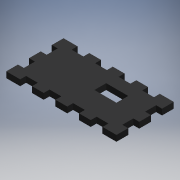
# Autodesk Inventor part: left
Saved by Autodesk Inventor 2019 (Build 230136000, 136)
## iProperties
Created: 2018-06-07
Part Number: left
Material: PBT Plastic Black
Document SubType Name: Modeling
Designer: stra92745
Density: 1.31 g/cm^3
Appearance: Smooth - White
Author: stra92745
Autodesk Inventor part; units mm, degrees
ref_plane "YZ Plane" through (0, 0, 0) normal (1, 0, 0) x (0, 1, 0)
ref_plane "XZ Plane" through (0, 0, 0) normal (0, 1, 0) x (-1, 0, 0)
ref_plane "XY Plane" through (0, 0, 0) normal (0, 0, 1) x (1, 0, 0)
sketch "Sketch1" plane through (0, 0, 0) normal (0, 1, 0) x (-1, 0, 0)
  line L0 (0, 0) -> (-75, 0)
  line L1 (-75, 0) -> (-75, -39)
  line L2 (-75, -39) -> (0, -39)
  line L3 (0, -39) -> (0, 0)
  line L4 (-41, -27) -> (-56, -27)
  line L5 (-56, -27) -> (-56, -19)
  line L6 (-56, -19) -> (-41, -19)
  line L7 (-41, -19) -> (-41, -27)
  dimension "d0" = 75
  dimension "d1" = 39
  dimension "d21" = 15
  dimension "d22" = 19
  dimension "d23" = 8
  dimension "d24" = 19
  constraints: 16 end point, 4 parallel, 2 horizontal, 2 perpendicular
  measures "d0" distance of L2.end L1.end
  measures "d1" distance of L1.end L0.end
  measures "d21" distance of L5.end L6.end
  measures "d22" distance between parallel lines of L1 L5
  measures "d23" distance of L6.end L4.start
  measures "d24" distance between parallel lines of L0 L6
extrude "Extrusion1" add sketch "Sketch1" along normal blind 4
sketch "Sketch2" plane through (0, 4, 0) normal (0, 1, 0) x (1, 0, 0)
  line L0 (0, 39) -> (0, 0) construction
  line L1 (75, 39) -> (0, 39) construction
  line L2 (75, 0) -> (75, 39) construction
  line L3 (0, 0) -> (75, 0) construction
  line L4 (4, 35) -> (4, 4) construction
  line L5 (4, 4) -> (71, 4) construction
  line L6 (71, 4) -> (71, 35) construction
  line L7 (71, 35) -> (4, 35) construction
  line L8 (0, 39) -> (0, 0) construction
  line L9 (0, 19.5) -> (75, 19.5) construction
  line L10 (37.5, 39) -> (37.5, 0) construction
  line L11 (0, 31) -> (4, 31)
  line L12 (4, 31) -> (4, 23.5)
  line L13 (4, 23.5) -> (0, 23.5)
  line L14 (0, 23.5) -> (0, 31)
  line L15 (75, 39) -> (0, 39) projected
  line L16 (9.5, 35) -> (17.5, 35)
  line L17 (17.5, 35) -> (17.5, 39)
  line L18 (17.5, 39) -> (9.5, 39)
  line L19 (9.5, 39) -> (9.5, 35)
  line L20 (25.5, 35) -> (33.5, 35)
  line L21 (33.5, 35) -> (33.5, 39)
  line L22 (33.5, 39) -> (25.5, 39)
  line L23 (25.5, 39) -> (25.5, 35)
  line L24 (75, 31) -> (71, 31)
  line L25 (71, 31) -> (71, 23.5)
  line L26 (71, 23.5) -> (75, 23.5)
  line L27 (75, 23.5) -> (75, 31)
  line L28 (65.5, 35) -> (57.5, 35)
  line L29 (57.5, 35) -> (57.5, 39)
  line L30 (57.5, 39) -> (65.5, 39)
  line L31 (65.5, 39) -> (65.5, 35)
  line L32 (49.5, 35) -> (41.5, 35)
  line L33 (41.5, 35) -> (41.5, 39)
  line L34 (41.5, 39) -> (49.5, 39)
  line L35 (49.5, 39) -> (49.5, 35)
  line L36 (75, 0) -> (0, 0) construction
  line L37 (71, 4) -> (4, 4) construction
  line L38 (0, 8) -> (4, 8)
  line L39 (4, 8) -> (4, 15.5)
  line L40 (4, 15.5) -> (0, 15.5)
  line L41 (0, 15.5) -> (0, 8)
  line L42 (75, 0) -> (0, 0)
  line L43 (9.5, 4) -> (17.5, 4)
  line L44 (17.5, 4) -> (17.5, 0)
  line L45 (17.5, 0) -> (9.5, 0)
  line L46 (9.5, 0) -> (9.5, 4)
  line L47 (25.5, 4) -> (33.5, 4)
  line L48 (33.5, 4) -> (33.5, 0)
  line L49 (33.5, 0) -> (25.5, 0)
  line L50 (25.5, 0) -> (25.5, 4)
  line L51 (49.5, 4) -> (41.5, 4)
  line L52 (49.5, 0) -> (49.5, 4)
  line L53 (41.5, 0) -> (49.5, 0)
  line L54 (41.5, 4) -> (41.5, 0)
  line L55 (57.5, 4) -> (57.5, 0)
  line L56 (65.5, 4) -> (57.5, 4)
  line L57 (57.5, 0) -> (65.5, 0)
  line L58 (71, 8) -> (71, 15.5)
  line L59 (71, 15.5) -> (75, 15.5)
  line L60 (75, 15.5) -> (75, 8)
  line L61 (75, 8) -> (71, 8)
  line L62 (65.5, 0) -> (65.5, 4)
  dimension "d12" = 4
  dimension "d13" = 4
  dimension "d14" = 8
  dimension "d15" = 8
  dimension "d16" = 8
  dimension "d17" = 8
  dimension "d18" = 4
  constraints: 114 end point, 36 symmetric about line, 12 point on line, 4 midpoint, 4 parallel, 4 perpendicular, 2 horizontal, 1 collinear, 3 other
  measures "d12" distance between parallel lines of L1 L7
  measures "d13" distance between parallel lines of L9 L13
  measures "d14" distance between parallel lines of L11 L1
  measures "d15" distance of L20.start L20.end
  measures "d16" distance of L16.start L16.end
  measures "d17" distance between parallel lines of L23 L17
  measures "d18" distance between parallel lines of L10 L21
extrude "Extrusion2" cut sketch "Sketch2" against normal up to surface (4 mm away)
body "Solid1"
